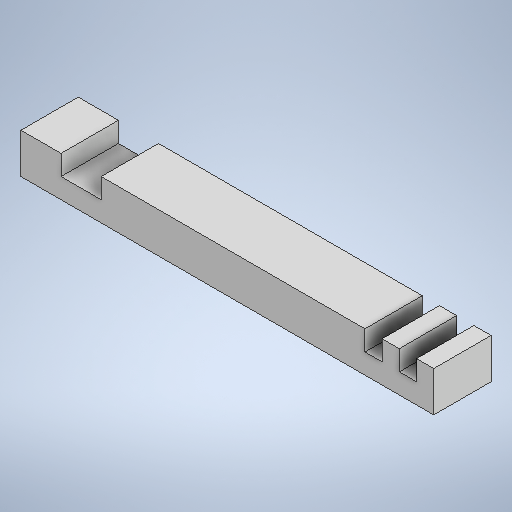
# Autodesk Inventor part: Wall Test
Saved by Autodesk Inventor 2025.2 (Build 292293000, 293)
## iProperties
Created: 2025-05-10
Part Number: Wall Test
Material: Generic
Document SubType Name: Modeling
Designer: powel
Density: 1 g/cm^3
Appearance: Default
Author: powel
Autodesk Inventor part; units mm, degrees
ref_plane "YZ Plane" through (0, 0, 0) normal (1, 0, 0) x (0, 1, 0)
ref_plane "XZ Plane" through (0, 0, 0) normal (0, 1, 0) x (-1, 0, 0)
ref_plane "XY Plane" through (0, 0, 0) normal (0, 0, 1) x (1, 0, 0)
sketch "Sketch1" plane through (0, 0, 0) normal (0, 1, 0) x (-1, 0, 0)
  line L0 (0, 0) -> (36, 0)
  line L1 (36, 0) -> (36, -5)
  line L2 (36, -5) -> (0, -5)
  line L3 (0, -5) -> (0, 0)
  line L4 (0, 0) -> (1.5, 0)
  line L5 (1.5, 0) -> (1.5, -5)
  line L6 (1.5, -5) -> (0, -5)
  line L7 (0, -5) -> (0, 0)
  line L8 (1.5, -5) -> (3, -5)
  line L9 (3, -5) -> (3, 0)
  line L10 (3, 0) -> (1.5, 0)
  line L11 (1.5, 0) -> (1.5, -5)
  line L12 (3, 0) -> (4.5, 0)
  line L13 (4.5, 0) -> (4.5, -5)
  line L14 (4.5, -5) -> (3, -5)
  line L15 (3, -5) -> (3, 0)
  line L16 (4.5, -5) -> (6, -5)
  line L17 (6, -5) -> (6, 0)
  line L18 (6, 0) -> (4.5, 0)
  line L19 (4.5, 0) -> (4.5, -5)
  line L20 (36, -5) -> (32.5, -5)
  line L21 (32.5, -5) -> (32.5, 0)
  line L22 (32.5, 0) -> (36, 0)
  line L23 (36, 0) -> (36, -5)
  line L24 (32.5, 0) -> (29, 0)
  line L25 (29, 0) -> (29, -5)
  line L26 (29, -5) -> (32.5, -5)
  line L27 (32.5, -5) -> (32.5, 0)
  dimension "d0" = 36
  dimension "d1" = 5
  dimension "d2" = 1.5
  dimension "d3" = 1.5
  dimension "d4" = 1.5
  dimension "d5" = 1.5
  dimension "d6" = 3.5
  dimension "d7" = 3.5
  constraints: 56 end point, 14 parallel, 7 horizontal, 7 perpendicular, 6 point on line
  measures "d0" distance of L1.end L2.end
  measures "d1" distance of L0.end L1.end
  measures "d2" distance of L5.end L6.end
  measures "d3" distance of L10.end L9.end
  measures "d4" distance of L13.end L14.end
  measures "d5" distance of L18.end L17.end
  measures "d6" distance of L21.end L22.end
  measures "d7" distance of L26.end L25.end
extrude "Extrusion1" add sketch "Sketch1" along normal blind 1.75 contours L0 L5 L2 L3 | L0 L13 L2 L9 | L0 L25 L2 L17 | L0 L1 L2 L21
extrude "Extrusion2" add sketch "Sketch1" against normal blind 1.75
body "Solid1"
